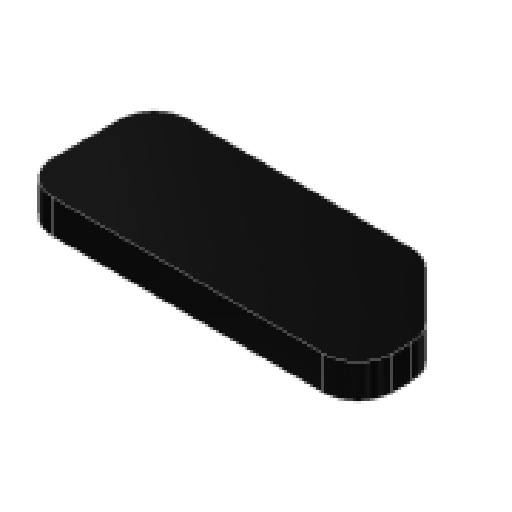
# Autodesk Inventor part: Frame_Foot_Flex
Saved by Autodesk Inventor 2023.2 (Build 272271000, 271)
## iProperties
Created: 2020-05-24
Part Number: Frame_Foot_Flex
Material: Rubber, Silicone
Document SubType Name: Modeling
Designer: Remo
Density: 1.25 g/cm^3
Appearance: Glossy - Black
Description: 3DP Part / Ninjaflex / Machine Foot - Dampener
Author: Remo
Revision Number: 1
Autodesk Inventor part; units mm, degrees
ref_plane "YZ Plane" through (0, 0, 0) normal (1, 0, 0) x (0, 1, 0)
ref_plane "XZ Plane" through (0, 0, 0) normal (0, 1, 0) x (-1, 0, 0)
ref_plane "XY Plane" through (0, 0, 0) normal (0, 0, 1) x (1, 0, 0)
sketch "Sketch1" plane through (0, 0, 0) normal (0, 0, 1) x (1, 0, 0)
  circle A0 centre (40, 19.5) radius 1.85 projected
  circle A1 centre (-57.5, -20.4606) radius 1.85 projected
  circle A2 centre (-57.5, 19.5) radius 1.85 projected
  circle A3 centre (57.5, -20.4606) radius 1.85 projected
  line L0 (63, 25) -> (-63, 25) projected
  line L1 (-63, 25) -> (-63, -25) projected
  line L2 (-63, -25) -> (63, -25) projected
  line L3 (63, -25) -> (63, 25) projected
  line L4 (50, -20) -> (-50, -20)
  line L5 (-50, -20) -> (-50, 20)
  line L6 (-50, 20) -> (50, 20)
  line L7 (50, 20) -> (50, -20)
  line L8 (50, -20) -> (-50, 20) construction
  line L9 (-50, -20) -> (50, 20) construction
  point P0 (0, 0)
  dimension "d0" = 40
  dimension "d1" = 100
  constraints: 12 end point, 2 midpoint, 2 parallel, 1 horizontal, 1 perpendicular
  measures "d0" distance of L4.end L5.end
  measures "d1" distance of L4.start L4.end
extrude "Extrusion1" add sketch "Sketch1" along normal blind 10 contours A0 L6 | A0 L6 L7 L4 L5 picked at (39.6393, 19.3331)
chamfer "Chamfer1" distance 20 angle 45 1 edges at (50, 20, 5)
fillet "Fillet1" radius 10 5 edges at (-50, 20, 5) (30, 20, 5) (50, 0, 5) (50, -20, 5) (-50, -20, 5)
body "Solid1"
